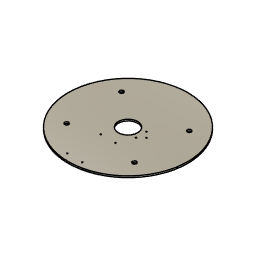
Turn Table Top (Autodesk Fusion 360 design; units mm, degrees)
Autodesk Fusion 360 part; units mm, degrees
sketch "スケッチ1" plane through (0, 0, 0) normal (0, 0, 1) x (1, 0, 0)
  line L0 (68, -55) -> (-68, -55)
  line L1 (-68, -55) -> (-68, 55)
  line L2 (-68, 55) -> (68, 55)
  line L3 (68, 55) -> (68, -55)
  line L4 (68, -55) -> (-68, 55) construction
  line L5 (-68, -55) -> (68, 55) construction
  circle A0 centre (-68, 55) radius 4.05
  circle A1 centre (68, 55) radius 4.05
  circle A2 centre (-68, -55) radius 4.05
  circle A3 centre (68, -55) radius 4.05
  circle A4 centre (0, 0) radius 35
  circle A5 centre (0, 0) radius 130
  dimension "d1" = 136
  dimension "d2" = 110
  dimension "d3" = 8.1
  dimension "d4" = 8.1
  dimension "d5" = 8.1
  dimension "d6" = 8.1
  dimension "d18" = 70
  dimension "d19" = 260
  constraint horizontal L0
  constraint perpendicular L0 L1
  constraint parallel L0 L2
  constraint parallel L1 L3
  constraint coincident L4 A4.centre
  constraint coincident L5 A4.centre
  constraint coincident A4.centre A5.centre
  constraint coincident L1.end L2.start
  constraint coincident L2.end L3.start
  constraint coincident L0.end L1.start
  constraint coincident L0.start L3.end
  measures "d1" distance of L1.end L2.end
  measures "d2" distance of L0.end L1.end
  measures "d3" diameter of A0
  measures "d4" diameter of A1
  measures "d5" diameter of A2
  measures "d6" diameter of A3
  measures "d18" diameter of A4
  measures "d19" diameter of A5
extrude "押し出し1" add sketch "スケッチ1" along normal blind 1 contours L0 L1 L2 L3 A0 A1 A2 A3 | A5
sketch "スケッチ7" plane through (0, 0, 1) normal (0, 0, 1) x (-1, 0, 0)
  circle A0 centre (68, -55) radius 4.05
  circle A1 centre (68, 55) radius 4.05
  circle A2 centre (-68, -55) radius 4.05
  circle A3 centre (-68, 55) radius 4.05
  circle A4 centre (0, 0) radius 35
  circle A5 centre (0, 0) radius 130
  circle A6 centre (0, 0) radius 25
  dimension "d809" = 50
  constraint concentric A4 A6
  measures "d809" diameter of A6
extrude "押し出し11" add sketch "スケッチ7" against normal blind 1 contours A4
sketch "スケッチ8" plane through (0, 0, 1) normal (0, 0, 1) x (-1, 0, 0)
  circle A0 centre (0, 0) radius 25
  circle A1 centre (68, -55) radius 4.05
  circle A2 centre (68, 55) radius 4.05
  circle A3 centre (-68, -55) radius 4.05
  circle A4 centre (-68, 55) radius 4.05
  circle A5 centre (0, 0) radius 130
  line L0 (0, 0) -> (16.5, 0)
  line L1 (16.5, 0) -> (16.5, 25.6)
  circle A6 centre (16.5, 25.6) radius 1.25
  line L2 (0, 0) -> (-16.5, 0)
  line L3 (-16.5, 0) -> (-16.5, -25.6)
  circle A7 centre (-16.5, -25.6) radius 1.25
  line L4 (-16.5, -25.6) -> (-37.5, -25.6)
  circle A8 centre (-37.5, -25.6) radius 1.25
  line L5 (-27, -25.6) -> (-27, -36.1)
  line L6 (-27, -25.6) -> (-27, -15.1)
  circle A9 centre (-27, -36.1) radius 1.25
  circle A10 centre (-27, -15.1) radius 1.25
  dimension "d812" = 16.5
  dimension "d813" = 25.6
  dimension "d814" = 2.5
  dimension "d817" = 16.5
  dimension "d818" = 25.6
  dimension "d819" = 2.5
  dimension "d822" = 21
  dimension "d823" = 2.5
  dimension "d824" = 10.5
  dimension "d825" = 10.5
  dimension "d826" = 2.5
  dimension "d827" = 2.5
  constraint coincident A0.centre A5.centre
  constraint horizontal L0
  constraint perpendicular L0 L1
  constraint coincident L1.end A6.centre
  constraint parallel L0 L2
  constraint perpendicular L2 L3
  constraint coincident L3.end A7.centre
  constraint perpendicular L3 L4
  constraint coincident L4.end A8.centre
  constraint midpoint L4 L5.start
  constraint perpendicular L4 L5
  constraint perpendicular L4 L6
  constraint coincident L5.end A9.centre
  constraint coincident L6.end A10.centre
  measures "d812" distance of A0.centre L0.end
  measures "d813" distance of L0.end L1.end
  measures "d814" diameter of A6
  measures "d817" distance of A0.centre L2.end
  measures "d818" distance of L2.end L3.end
  measures "d819" diameter of A7
  measures "d822" distance of L3.end L4.end
  measures "d823" diameter of A8
  measures "d824" distance of L5.start L5.end
  measures "d825" distance of L5.start L6.end
  measures "d826" diameter of A9
  measures "d827" diameter of A10
extrude "押し出し13" cut sketch "スケッチ8" against normal blind 1 contours L3 A7 L4 | L3 A7 L4 | A8 | A9 | A10
sketch "スケッチ9" plane through (0, 0, 1) normal (0, 0, 1) x (-1, 0, 0)
  circle A0 centre (-27, -36.1) radius 1.25
  circle A1 centre (-37.5, -25.6) radius 1.25
  circle A2 centre (-16.5, -25.6) radius 1.25
  circle A3 centre (-27, -15.1) radius 1.25
  circle A4 centre (0, 0) radius 25
  circle A5 centre (68, -55) radius 4.05
  circle A6 centre (68, 55) radius 4.05
  circle A7 centre (-68, -55) radius 4.05
  circle A8 centre (-68, 55) radius 4.05
  circle A9 centre (0, 0) radius 130
  circle A10 centre (0, 0) radius 120
  dimension "d828" = -10
extrude "押し出し14" cut sketch "スケッチ9" against normal blind 1 contours A9
sketch "スケッチ10" plane through (0, 0, 1) normal (0, 0, 1) x (-1, 0, 0)
  circle A0 centre (0, 0) radius 120
  circle A1 centre (-27, -36.1) radius 1.25
  circle A2 centre (-37.5, -25.6) radius 1.25
  circle A3 centre (-16.5, -25.6) radius 1.25
  circle A4 centre (-27, -15.1) radius 1.25
  circle A5 centre (0, 0) radius 25
  circle A6 centre (68, -55) radius 4.05
  circle A7 centre (68, 55) radius 4.05
  circle A8 centre (-68, -55) radius 4.05
  circle A9 centre (-68, 55) radius 4.05
  line L0 (0, 0) -> (0, 40)
  line L1 (0, 40) -> (-15, 40)
  line L2 (0, 40) -> (15, 40)
  circle A10 centre (15, 40) radius 1.25
  circle A11 centre (-15, 40) radius 1.25
  dimension "d838" = 40
  dimension "d839" = 15
  dimension "d840" = 15
  dimension "d841" = 2.5
  dimension "d842" = 2.5
  constraint coincident A0.centre A5.centre
  constraint vertical L0
  constraint perpendicular L0 L1
  constraint perpendicular L0 L2
  constraint coincident L2.end A10.centre
  constraint coincident L1.end A11.centre
  measures "d838" distance of A0.centre L0.end
  measures "d839" distance of L0.end L1.end
  measures "d840" distance of L0.end L2.end
  measures "d841" diameter of A10
  measures "d842" diameter of A11
extrude "押し出し16" cut sketch "スケッチ10" against normal blind 1 contours A10 | A11
sketch "スケッチ11" plane through (0, 0, 1) normal (0, 0, 1) x (-1, 0, 0)
  circle A0 centre (-15, 40) radius 1.25
  circle A1 centre (15, 40) radius 1.25
  circle A2 centre (0, 0) radius 120
  circle A3 centre (-27, -36.1) radius 1.25
  circle A4 centre (-37.5, -25.6) radius 1.25
  circle A5 centre (-16.5, -25.6) radius 1.25
  circle A6 centre (-27, -15.1) radius 1.25
  circle A7 centre (0, 0) radius 25
  circle A8 centre (68, -55) radius 4.05
  circle A9 centre (68, 55) radius 4.05
  circle A10 centre (-68, -55) radius 4.05
  circle A11 centre (-68, 55) radius 4.05
  line L0 (0, 0) -> (0, 107)
  line L1 (0, 107) -> (15, 107)
  line L2 (0, 107) -> (-15, 107)
  circle A12 centre (15, 107) radius 1.25
  circle A13 centre (-15, 107) radius 1.25
  dimension "d845" = 107
  dimension "d846" = 15
  dimension "d847" = 15
  dimension "d848" = 2.5
  dimension "d849" = 2.5
  constraint coincident A2.centre A7.centre
  constraint vertical L0
  constraint perpendicular L0 L1
  constraint perpendicular L0 L2
  constraint coincident L1.end A12.centre
  constraint coincident L2.end A13.centre
  measures "d845" distance of A2.centre L0.end
  measures "d846" distance of L0.end L1.end
  measures "d847" distance of L0.end L2.end
  measures "d848" diameter of A12
  measures "d849" diameter of A13
extrude "押し出し17" cut sketch "スケッチ11" against normal blind 1 contours A12 | A13
sketch "スケッチ12" plane through (0, 0, 1) normal (0, 0, 1) x (-1, 0, 0)
  circle A0 centre (15, 107) radius 1.25
  circle A1 centre (-15, 107) radius 1.25
  circle A2 centre (-15, 40) radius 1.25
  circle A3 centre (15, 40) radius 1.25
  circle A4 centre (0, 0) radius 120
  circle A5 centre (-27, -36.1) radius 1.25
  circle A6 centre (-37.5, -25.6) radius 1.25
  circle A7 centre (-16.5, -25.6) radius 1.25
  circle A8 centre (-27, -15.1) radius 1.25
  circle A9 centre (0, 0) radius 25
  circle A10 centre (68, -55) radius 4.05
  circle A11 centre (68, 55) radius 4.05
  circle A12 centre (-68, -55) radius 4.05
  circle A13 centre (-68, 55) radius 4.05
  line L0 (-37.5, -25.6) -> (-37.5, 0)
  circle A14 centre (-37.5, 0) radius 1.25
  line L1 (-27, -15.1) -> (-27, 10.5)
  circle A15 centre (-27, 10.5) radius 1.25
  line L2 (-27, -36.1) -> (-27, -10.5)
  circle A16 centre (-27, -10.5) radius 1.25
  dimension "d852" = 25.6
  dimension "d853" = 2.5
  dimension "d854" = 25.6
  dimension "d855" = 2.5
  dimension "d856" = 25.6
  dimension "d857" = 2.5
  constraint coincident A6.centre L0.start
  constraint vertical L0
  constraint coincident L0.end A14.centre
  constraint coincident A8.centre L1.start
  constraint vertical L1
  constraint coincident L1.end A15.centre
  constraint coincident A5.centre L2.start
  constraint vertical L2
  constraint coincident L2.end A16.centre
  measures "d852" distance of A6.centre L0.end
  measures "d853" diameter of A14
  measures "d854" distance of A8.centre L1.end
  measures "d855" diameter of A15
  measures "d856" distance of A5.centre L2.end
  measures "d857" diameter of A16
extrude "押し出し18" add sketch "スケッチ12" against normal blind 1 contours A5 | A6 | A7 | A8 L1 L2 | A8 L1 L2
extrude "押し出し19" cut sketch "スケッチ12" against normal blind 1 contours A14 | L1 L2 A16 | L1 L2 A16 | A15
extrude "押し出し20" add 1 faces at (-71.1115, -16.9879, 0) along direction (0, 0, -1) blind 2
sketch "スケッチ13" plane through (0, 0, 1) normal (0, 0, 1) x (-1, 0, 0)
  circle A0 centre (-37.5, 0) radius 1.25
  circle A1 centre (-27, 10.5) radius 1.25
  circle A2 centre (-27, -10.5) radius 1.25
  circle A3 centre (15, 107) radius 1.25
  circle A4 centre (-15, 107) radius 1.25
  circle A5 centre (-15, 40) radius 1.25
  circle A6 centre (15, 40) radius 1.25
  circle A7 centre (0, 0) radius 120
  circle A8 centre (0, 0) radius 25
  circle A9 centre (68, -55) radius 4.05
  circle A10 centre (68, 55) radius 4.05
  circle A11 centre (-68, -55) radius 4.05
  circle A12 centre (-68, 55) radius 4.05
  circle A13 centre (0, 0) radius 20
  dimension "d864" = 40
  constraint concentric A7 A13
  measures "d864" diameter of A13
extrude "押し出し21" add sketch "スケッチ13" against normal blind 3 contours A8
sketch "スケッチ14" plane through (0, 0, 1) normal (0, 0, 1) x (-1, 0, 0)
  circle A0 centre (0, 0) radius 20
  circle A1 centre (-37.5, 0) radius 1.25
  circle A2 centre (-27, 10.5) radius 1.25
  circle A3 centre (-27, -10.5) radius 1.25
  circle A4 centre (15, 107) radius 1.25
  circle A5 centre (-15, 107) radius 1.25
  circle A6 centre (-15, 40) radius 1.25
  circle A7 centre (15, 40) radius 1.25
  circle A8 centre (0, 0) radius 120
  circle A9 centre (68, -55) radius 4.05
  circle A10 centre (68, 55) radius 4.05
  circle A11 centre (-68, -55) radius 4.05
  circle A12 centre (-68, 55) radius 4.05
  line L0 (-37.5, 0) -> (-37, 0)
  line L1 (-27, -10.5) -> (-26.5, -10.5)
  line L2 (-27, 10.5) -> (-26.5, 10.5)
  circle A13 centre (-26.5, -10.5) radius 1.25
  circle A14 centre (-37, 0) radius 1.25
  circle A15 centre (-26.5, 10.5) radius 1.25
  dimension "d867" = 0.5
  dimension "d868" = 0.5
  dimension "d869" = 0.5
  dimension "d870" = 2.5
  dimension "d871" = 2.5
  dimension "d872" = 2.5
  constraint coincident A1.centre L0.start
  constraint horizontal L0
  constraint coincident A3.centre L1.start
  constraint horizontal L1
  constraint coincident A2.centre L2.start
  constraint horizontal L2
  constraint coincident L1.end A13.centre
  constraint coincident L0.end A14.centre
  constraint coincident L2.end A15.centre
  measures "d867" distance of A1.centre L0.end
  measures "d868" distance of A3.centre L1.end
  measures "d869" distance of A2.centre L2.end
  measures "d870" diameter of A13
  measures "d871" diameter of A14
  measures "d872" diameter of A15
extrude "押し出し22" cut sketch "スケッチ14" against normal blind 3 contours A1 A14 | A2 A15 | A3 A13 picked at (-35.9431, -0.2395) picked at (-25.4431, 10.2605) picked at (-25.4431, -10.7395)
extrude "押し出し23" add sketch "スケッチ14" against normal blind 3 contours A1 A14 | A2 A15 | A3 A13 picked at (-38.5777, -0.0913) picked at (-28.0777, 10.5913) picked at (-28.0777, -10.4087)
sketch "スケッチ15" plane through (0, 0, 1) normal (0, 0, 1) x (-1, 0, 0)
  circle A0 centre (-68, 55) radius 4.05
  circle A1 centre (-68, -55) radius 4.05
  circle A2 centre (68, 55) radius 4.05
  circle A3 centre (68, -55) radius 4.05
  circle A4 centre (0, 0) radius 120
  circle A5 centre (15, 40) radius 1.25
  circle A6 centre (-15, 40) radius 1.25
  circle A7 centre (-15, 107) radius 1.25
  circle A8 centre (15, 107) radius 1.25
  circle A9 centre (-26.5, -10.5) radius 1.25
  circle A10 centre (-26.5, 10.5) radius 1.25
  circle A11 centre (-37, 0) radius 1.25
  circle A12 centre (0, 0) radius 20
  circle A13 centre (0, 0) radius 19.5
  dimension "d877" = 39
  constraint concentric A4 A13
  measures "d877" diameter of A13
extrude "押し出し24" add sketch "スケッチ15" against normal blind 3 contours A12
